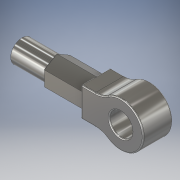
# Autodesk Inventor part: Single Eye End
Saved by Autodesk Inventor 2018 (Build 220112000, 112)
## iProperties
Created: 2019-09-01
Part Number: Single Eye End
Material: Generic
Document SubType Name: Modeling
Designer: Sameer
Density: 1 g/cm^3
Appearance: Chrome - Polished
Author: Sameer
Autodesk Inventor part; units mm, degrees
ref_plane "YZ Plane" through (0, 0, 0) normal (1, 0, 0) x (0, 1, 0)
ref_plane "XZ Plane" through (0, 0, 0) normal (0, 1, 0) x (-1, 0, 0)
ref_plane "XY Plane" through (0, 0, 0) normal (0, 0, 1) x (1, 0, 0)
sketch "Sketch1" plane through (0, 0, 0) normal (0, 0, 1) x (1, 0, 0)
  line L0 (-17.5, 13) -> (2.3013, 13)
  line L1 (2.3013, -13) -> (-17.5, -13)
  line L2 (-17.5, -13) -> (-17.5, 13)
  arc A0 (2.3013, -13) -> (2.3013, 13) centre (17.5, 0) ccw
  circle A1 centre (17.5, 0) radius 10
  point P0 (0, 0)
  constraints: 6 end point, 2 centre point, 2 point on circle, 1 coincident, 1 horizontal, 1 parallel
extrude "Extrusion1" add sketch "Sketch1" along normal mid plane 26
sketch "Sketch2" plane through (-17.5, -13, 13) normal (-1, 0, 0) x (0, 0, 1)
  line L0 (-26, 26) -> (0, 26) projected
  line L1 (-13, 26) -> (-1.7417, 19.5)
  line L2 (-1.7417, 19.5) -> (-1.7417, 6.5)
  line L3 (-1.7417, 6.5) -> (-13, 0)
  line L4 (-13, 0) -> (-24.2583, 6.5)
  line L5 (-24.2583, 6.5) -> (-24.2583, 19.5)
  line L6 (-24.2583, 19.5) -> (-13, 26)
  point P0 (-13, 13)
  point P1 (-13, 13)
  constraints: 12 end point, 1 coincident, 1 midpoint, 13 other
extrude "Extrusion2" add sketch "Sketch2" along normal blind 35
sketch "Sketch3" plane through (-52.5, -13, 13) normal (-1, 0, 0) x (0, 0, 1)
  circle A0 centre (-13, 13) radius 10
  constraints: 1 centre point, 1 coincident
extrude "Extrusion3" add sketch "Sketch3" along normal blind 30
fillet "Fillet1" radius 20 1 edges at (2.3013, 13, 0)
fillet "Fillet2" radius 20 1 edges at (2.3013, -13, 0)
chamfer "Chamfer1" distance 1 angle 45 6 edges at (-52.5, -9.75, -5.6292) (-52.5, 0, -11.2583) (-52.5, 9.75, -5.6292) (-52.5, -9.75, 5.6292) (-52.5, 0, 11.2583) (-52.5, 9.75, 5.6292)
fillet "Fillet3" radius 1 18 edges at (7.5, 0, -13) (7.5, 0, 13) (0.8108, -13.895, -13) (-11.3027, -13, -13) (0.8108, 13.895, -13) (-11.3027, 13, -13) (37.5, 0, -13) (-17.5, 0, -13) (0.8108, -13.895, 13) (37.5, 0, 13) (0.8108, 13.895, 13) (-11.3027, 13, 13) (-11.3027, -13, 13) (-17.5, 0, 13) (-17.5, -13, 6.5) (-17.5, -13, -6.5) (-17.5, 13, 6.5) (-17.5, 13, -6.5)
body "Solid1"
